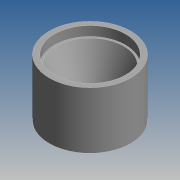
# Autodesk Inventor part: P009_CanonAdaptateurReservoir
Saved by Autodesk Inventor 2020 (Build 240168000, 168)
## iProperties
Created: 2021-10-15
Part Number: P009_CanonAdaptateurReservoir
Material: Générique
Document SubType Name: Modeling
Designer: gabri
Density: 1 g/cm^3
Appearance: Par défaut
Author: gabri
Autodesk Inventor part; units mm, degrees
ref_plane "YZ Plane" through (0, 0, 0) normal (1, 0, 0) x (0, 1, 0)
ref_plane "XZ Plane" through (0, 0, 0) normal (0, 1, 0) x (-1, 0, 0)
ref_plane "XY Plane" through (0, 0, 0) normal (0, 0, 1) x (1, 0, 0)
sketch "Esquisse2" plane through (0, 0, 0) normal (0, 1, 0) x (-1, 0, 0)
  line L0 (0, 0) -> (0, 53.3255)
  line L1 (-15, 5) -> (-18, 5)
  line L2 (-18, 5) -> (-18, 10)
  line L3 (8.6, 0) -> (-51.6, 0) construction
  line L4 (-15, 5) -> (-15, 14.8264)
  line L5 (-15, 14.8264) -> (-35.5, 60)
  line L6 (-35.5, 60) -> (-37.5, 60)
  line L7 (-37.5, 60) -> (-37.5, 70)
  line L8 (-37.5, 70) -> (-43, 70)
  line L9 (-18, 10) -> (-43, 10)
  line L10 (-43, 10) -> (-43, 70)
  dimension "d0" = 36
  dimension "d2" = 3
  dimension "d3" = 30
  dimension "d4" = 75
  dimension "d6" = 86
  dimension "d7" = 60
  dimension "d8" = 10
  dimension "d9" = 5
  dimension "d10" = 2
  dimension "d11" = 50
  dimension "d12" = 24.409
  constraints: 20 end point, 3 horizontal, 3 perpendicular, 2 vertical, 1 parallel
  measures "d0" diameter of L2 L0
  measures "d2" distance of L1.start L1.end
  measures "d3" diameter of L4 L0
  measures "d4" diameter of L7 L0
  measures "d6" diameter of L10 L0
  measures "d7" distance between parallel lines of L8 L9
  measures "d8" distance between parallel lines of L3 L9
  measures "d9" distance of L1.end L2.end
  measures "d10" distance of L5.end L6.end
  measures "d11" distance between parallel lines of L9 L6
  measures "d12" angle of L0 L5
revolve "Révolution1" add sketch "Esquisse2" angle 360 about axis through (0, 0, 0) along (0, 0, 1)
